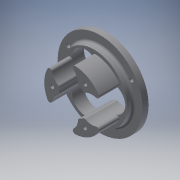
# Autodesk Inventor part: LayerBase1
Saved by Autodesk Inventor 2019 (Build 230136000, 136)
## iProperties
Created: 2022-08-24
Part Number: LayerBase1
Material: Generic
Document SubType Name: Modeling
Designer: zreik
Density: 1 g/cm^3
Appearance: Default
Author: zreik
Autodesk Inventor part; units mm, degrees
ref_plane "YZ Plane" through (0, 0, 0) normal (1, 0, 0) x (0, 1, 0)
ref_plane "XZ Plane" through (0, 0, 0) normal (0, 1, 0) x (-1, 0, 0)
ref_plane "XY Plane" through (0, 0, 0) normal (0, 0, 1) x (1, 0, 0)
sketch "Sketch1" plane through (0, 0, 0) normal (0, 0, 1) x (1, 0, 0)
  circle A0 centre (0, 0) radius 35.5
  circle A1 centre (0, 0) radius 12.5
  dimension "d0" = 71
  dimension "d1" = 25
  constraints: 2 centre point, 2 coincident
  measures "d0" diameter of A0
  measures "d1" diameter of A1
extrude "Extrusion1" add sketch "Sketch1" along normal blind 27
sketch "Sketch2" plane through (0, 0, 27) normal (0, 0, 1) x (1, 0, 0)
  circle A0 centre (0, 0) radius 24.75
  circle A1 centre (0, 0) radius 35.5
  dimension "d4" = 71
  dimension "d5" = 49.5
  constraints: 2 centre point, 2 coincident
  measures "d4" diameter of A1
  measures "d5" diameter of A0
extrude "Extrusion2" cut sketch "Sketch2" against normal blind 22
sketch "Sketch3" plane through (0, 0, 5) normal (0, 0, 1) x (1, 0, 0)
  circle A0 centre (0, 0) radius 27.5
  circle A1 centre (0, 0) radius 24.75
  dimension "d8" = 55
  dimension "d9" = 49.5
  constraints: 2 centre point, 2 coincident
  measures "d8" diameter of A0
  measures "d9" diameter of A1
extrude "Extrusion3" add sketch "Sketch3" along normal blind 5
fillet "Fillet1" radius 2 1 edges at (-27.5, 0, 5)
sketch "Sketch4" plane through (0, 0, 5) normal (0, 0, 1) x (1, 0, 0)
  circle A0 centre (26, 16) radius 1.75
  point P0 (0, 0)
  dimension "d13" = 3.5
  dimension "d14" = 26
  dimension "d15" = 16
  constraints: 1 centre point
  measures "d13" diameter of A0
  measures "d14" horizontal distance of point (0, 0) A0.centre
  measures "d15" vertical distance of point (0, 0) A0.centre
extrude "Extrusion4" cut sketch "Sketch4" along normal through all both and the other way through all
pattern_circular "Circular Pattern1" count 3 over 360 about axis through (0, 0, 7) along (0, 0, -1) of "Extrusion4"
sketch "Sketch5" plane through (0, 0, 27) normal (0, 0, 1) x (1, 0, 0)
  circle A0 centre (15, 0) radius 11
  point P0 (0, 0)
  dimension "d21" = 15
  dimension "d22" = 0
  dimension "d23" = 22
  constraints: 1 centre point
  measures "d21" distance of point (0, 0) A0.centre
  measures "d22" vertical distance of point (0, 0) A0.centre
  measures "d23" diameter of A0
extrude "Extrusion5" cut sketch "Sketch5" against normal up to next
fillet "Fillet2" radius 2 4 edges at (23.8854, -6.4845, 18.5) (23.8854, 6.4845, 18.5) (8.675, -8.9997, 13.5) (8.675, 8.9997, 13.5)
pattern_circular "Circular Pattern2" count 3 over 360 about axis through (0, 0, 27) along (0, 0, -1) of "Extrusion5", "Fillet2"
sketch "Sketch6" plane through (0, 0, 0) normal (0, 0, -1) x (-1, 0, 0)
  circle A0 centre (-9, -16) radius 1.75
  line L0 (-5.7668, -16) -> (-7.3834, -18.8)
  line L1 (-7.3834, -18.8) -> (-10.6166, -18.8)
  line L2 (-10.6166, -18.8) -> (-12.2332, -16)
  line L3 (-12.2332, -16) -> (-10.6166, -13.2)
  line L4 (-10.6166, -13.2) -> (-7.3834, -13.2)
  line L5 (-7.3834, -13.2) -> (-5.7668, -16)
  line L6 (49.7, 0) -> (-49.7, 0) projected
  point P0 (0, 0)
  dimension "d30" = 3.5
  dimension "d31" = 5.6
  dimension "d32" = 16
  dimension "d33" = 9
  constraints: 12 end point, 1 centre point, 1 coincident, 1 parallel, 13 other
  measures "d30" diameter of A0
  measures "d31" distance between parallel lines of L2 L5
  measures "d32" vertical distance of point (0, 0) A0.centre
  measures "d33" horizontal distance of point (0, 0) A0.centre
extrude "Extrusion6" cut sketch "Sketch6" against normal through all contours A0
extrude "Extrusion7" cut sketch "Sketch6" against normal blind 3
pattern_circular "Circular Pattern3" count 3 over 360 about axis through (0, 0, 0) along (0, 0, 1) of "Extrusion7", "Extrusion6"
body "Solid1"
